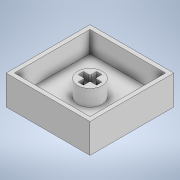
# Autodesk Inventor part: test2
Saved by Autodesk Inventor 2021.1 (Build 251245000, 245)
## iProperties
Created: 2020-08-05
Part Number: test2
Material: Generic
Document SubType Name: Modeling
Designer: adick
Density: 1 g/cm^3
Appearance: Default
Author: adick
Autodesk Inventor part; units mm, degrees
ref_plane "YZ Plane" through (0, 0, 0) normal (1, 0, 0) x (0, 1, 0)
ref_plane "XZ Plane" through (0, 0, 0) normal (0, 1, 0) x (-1, 0, 0)
ref_plane "XY Plane" through (0, 0, 0) normal (0, 0, 1) x (1, 0, 0)
sketch "Sketch1" plane through (0, 0, 0) normal (0, 1, 0) x (-1, 0, 0)
  line L0 (-10, 10) -> (10, 10)
  line L1 (10, 10) -> (10, -10)
  line L2 (10, -10) -> (-10, -10)
  line L3 (-10, -10) -> (-10, 10)
  line L4 (-10, 10) -> (10, -10) construction
  line L5 (10, 10) -> (-10, -10) construction
  point P0 (0, 0)
  constraints: 12 end point, 2 midpoint, 2 parallel, 1 horizontal, 1 perpendicular
extrude "Extrusion1" add sketch "Sketch1" along normal blind 2
sketch "Sketch2" plane through (0, 2, 0) normal (0, 1, 0) x (1, 0, 0)
  line L0 (9, -9) -> (-9, -9)
  line L1 (-9, -9) -> (-9, 9)
  line L2 (-9, 9) -> (9, 9)
  line L3 (9, 9) -> (9, -9)
  line L4 (9, -9) -> (-9, 9) construction
  line L5 (-9, -9) -> (9, 9) construction
  line L6 (10, -10) -> (-10, -10)
  line L7 (-10, -10) -> (-10, 10)
  line L8 (-10, 10) -> (10, 10)
  line L9 (10, 10) -> (10, -10)
  line L10 (10, -10) -> (-10, 10) construction
  line L11 (-10, -10) -> (10, 10) construction
  point P0 (0, 0)
  constraints: 24 end point, 4 midpoint, 4 parallel, 2 horizontal, 2 perpendicular, 1 point on line
extrude "Extrusion2" add sketch "Sketch2" along normal blind 5
sketch "Sketch3" plane through (0, 2, 0) normal (0, 1, 0) x (1, 0, 0)
  circle A0 centre (0, 0) radius 2.9425
  line L0 (0.626, -2.1935) -> (-0.626, -2.1935)
  line L1 (-0.626, 2.1935) -> (0.626, 2.1935)
  line L2 (-2.1935, 0.626) -> (-2.1935, -0.626)
  line L3 (2.1935, -0.626) -> (2.1935, 0.626)
  line L4 (-0.626, -2.1935) -> (-0.626, -0.626)
  line L5 (-0.626, 0.626) -> (-0.626, 2.1935)
  line L6 (-2.1935, -0.626) -> (-0.626, -0.626)
  line L7 (0.626, -0.626) -> (2.1935, -0.626)
  line L8 (2.1935, 0.626) -> (0.626, 0.626)
  line L9 (-0.626, 0.626) -> (-2.1935, 0.626)
  line L10 (0.626, 2.1935) -> (0.626, 0.626)
  line L11 (0.626, -0.626) -> (0.626, -2.1935)
  constraints: 24 end point, 10 parallel, 4 perpendicular, 3 horizontal, 1 centre point, 1 coincident
extrude "Extrusion4" add sketch "Sketch3" along normal blind 3.9
fillet "Fillet1" radius 0.3 4 edges at (-0.626, 3.95, -0.626) (-0.626, 3.95, 0.626) (0.626, 3.95, -0.626) (0.626, 3.95, 0.626)
body "Solid1"
